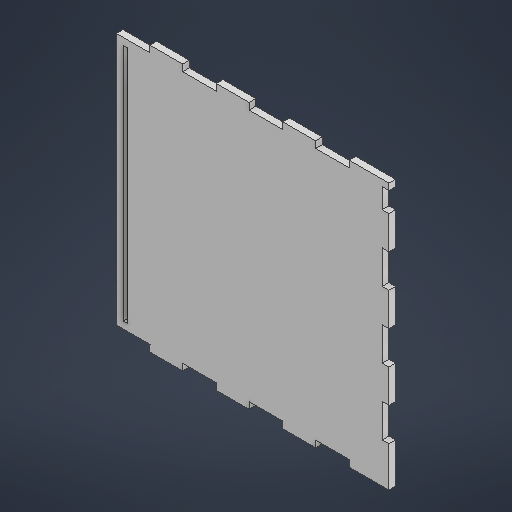
# Autodesk Inventor part: Base
Saved by Autodesk Inventor 2026 (Build 300175050, 175E)
## iProperties
Created: 2025-08-08
Part Number: Base
Material: Genérico
Document SubType Name: Modeling
Designer: EspacoMaker
Density: 1 g/cm^3
Appearance: Padrão
Author: EspacoMaker
Autodesk Inventor part; units mm, degrees
ref_plane "YZ Plane" through (0, 0, 0) normal (1, 0, 0) x (0, 1, 0)
ref_plane "XZ Plane" through (0, 0, 0) normal (0, 1, 0) x (-1, 0, 0)
ref_plane "XY Plane" through (0, 0, 0) normal (0, 0, 1) x (1, 0, 0)
sketch "Esboço1" plane through (0, 0, 0) normal (0, 0, 1) x (1, 0, 0)
  line L0 (-60, -60) -> (60, -60)
  line L1 (60, -60) -> (60, 60)
  line L2 (60, 60) -> (-60, 60)
  line L3 (-60, 60) -> (-60, -60)
  line L4 (-60, -60) -> (60, 60) construction
  line L5 (60, -60) -> (-60, 60) construction
  point P0 (0, 0)
  dimension "d0" = 120
  dimension "d1" = 120
  constraints: 12 end point, 2 midpoint, 2 parallel, 1 horizontal, 1 perpendicular
  measures "d0" distance of L2.end L1.end
  measures "d1" distance of L1.end L0.end
extrude "Extrusão1" add sketch "Esboço1" along normal blind 3
sketch "Esboço2" plane through (-60, 60, 0) normal (0, 1, 0) x (1, 0, 0)
  line L0 (120, -3) -> (0, -3) projected
  line L1 (120, 0) -> (0, 0) projected
  line L2 (0, -3) -> (15.1, -3)
  line L3 (15.1, -3) -> (15.1, 0)
  line L4 (15.1, 0) -> (0, 0)
  line L5 (0, 0) -> (0, -3)
  line L6 (-0.1, 0) -> (-0.1, -3)
  line L7 (29.9, 0) -> (29.9, -3)
  line L8 (45.1, 0) -> (30, 0)
  line L9 (30, -3) -> (45.1, -3)
  line L10 (45.1, -3) -> (45.1, 0)
  line L11 (59.9, 0) -> (59.9, -3)
  line L12 (75.1, 0) -> (60, 0)
  line L13 (60, -3) -> (75.1, -3)
  line L14 (75.1, -3) -> (75.1, 0)
  line L15 (89.9, 0) -> (89.9, -3)
  line L16 (105.1, 0) -> (90, 0)
  line L17 (90, -3) -> (105.1, -3)
  line L18 (105.1, -3) -> (105.1, 0)
  point P0 (89.9, 0)
  point P1 (59.9, 0)
  point P2 (29.9, 0)
  dimension "d4" = 15.1
  dimension "d57" = 30
  dimension "d63" = 0.1
  constraints: 34 end point, 9 point on line, 2 horizontal, 2 parallel, 2 perpendicular, 30 other
  measures "d4" distance of L4.end L3.end
  measures "d57" distance of L6.start L7.start
  measures "d63" distance between parallel lines of L6 L5
extrude "Extrusão2" cut sketch "Esboço2" against normal blind 3 contours L0 L15 L1 L18 | L0 L11 L1 L14 | L0 L7 L1 L10 | L0 L5 L1 L3
sketch "Esboço3" plane through (-60, -60, 0) normal (0, -1, 0) x (1, 0, 0)
  line L0 (0, 0) -> (120, 0) projected
  line L1 (0, 3) -> (15.1, 3)
  line L2 (15.1, 3) -> (15.1, 0)
  line L3 (15.1, 0) -> (0, 0)
  line L4 (0, 0) -> (0, 3)
  line L5 (-0.1, 0) -> (-0.1, 3)
  line L6 (-0.1, 0) -> (15.1, 0)
  line L7 (15.1, 0) -> (15.1, 3)
  line L8 (15.1, 3) -> (-0.1, 3)
  line L9 (-0.1, 3) -> (-0.1, 0)
  line L10 (29.9, 0) -> (29.9, 3)
  line L11 (45.1, 0) -> (30, 0)
  line L12 (30, 3) -> (45.1, 3)
  line L13 (45.1, 3) -> (45.1, 0)
  line L14 (59.9, 0) -> (59.9, 3)
  line L15 (75.1, 0) -> (60, 0)
  line L16 (60, 3) -> (75.1, 3)
  line L17 (75.1, 3) -> (75.1, 0)
  line L18 (89.9, 0) -> (89.9, 3)
  line L19 (105.1, 0) -> (90, 0)
  line L20 (90, 3) -> (105.1, 3)
  line L21 (105.1, 3) -> (105.1, 0)
  line L22 (0, 0) -> (0, 3) projected
  line L23 (0, 3) -> (120, 3) projected
  line L24 (120, 3) -> (120, 0) projected
  line L25 (120, 0) -> (0, 0) projected
  point P0 (-0.1, 1.5)
  point P1 (29.9, 1.5)
  point P2 (59.9, 1.5)
  point P3 (89.9, 1.5)
  point P4 (105.1, 0)
  point P5 (89.9, 0)
  point P6 (75.1, 0)
  point P7 (59.9, 0)
  point P8 (45.1, 0)
  point P9 (29.9, 0)
  dimension "d14" = 15.1
  dimension "d47" = 15.2
  dimension "d50" = 30
  dimension "d64" = 0.1
  constraints: 42 end point, 9 point on line, 4 parallel, 3 horizontal, 3 perpendicular, 1 collinear, 1 midpoint, 34 other
  measures "d14" distance of L2.end L3.end
  measures "d47" distance of L8.end L1.end
  measures "d50" distance of L5.start L10.start
  measures "d64" distance between parallel lines of L5 L4
extrude "Extrusão3" cut sketch "Esboço3" against normal blind 3 contours L4 L1 L2 L0 | L10 L23 L12 L13 L0 | L14 L23 L16 L17 L0 | L18 L23 L20 L21 L0
sketch "Esboço5" plane through (60, -60, 0) normal (1, 0, 0) x (0, 0, -1)
  line L0 (0, 3) -> (-3, 3) projected
  line L1 (-3, 3) -> (0, 3)
  line L2 (0, 3) -> (0, 18.1)
  line L3 (0, 18.1) -> (-3, 18.1)
  line L4 (-3, 18.1) -> (-3, 3)
  line L5 (0, 0) -> (-3, 0) projected
  line L6 (-3, 0) -> (-3, 120) projected
  line L7 (-3, 120) -> (0, 120) projected
  line L8 (0, 120) -> (0, 0) projected
  line L9 (0, 0) -> (-3, 0) projected
  line L10 (-3, 0) -> (-3, 120) projected
  line L11 (-3, 120) -> (0, 120) projected
  line L12 (0, 120) -> (0, 0) projected
  line L13 (-3, 3.1) -> (0, 3.1)
  line L14 (-3, 33.1) -> (0, 33.1)
  line L15 (0, 48.1) -> (-3, 48.1)
  line L16 (-3, 63.1) -> (0, 63.1)
  line L17 (0, 78.1) -> (-3, 78.1)
  line L18 (-3, 93.1) -> (0, 93.1)
  line L19 (0, 108.1) -> (-3, 108.1)
  line L20 (-3, 123.1) -> (0, 123.1)
  line L21 (0, 138.1) -> (-3, 138.1)
  line L22 (-3, 153.1) -> (0, 153.1)
  line L23 (0, 168.1) -> (-3, 168.1)
  line L24 (-3, 183.1) -> (0, 183.1)
  line L25 (0, 198.1) -> (-3, 198.1)
  line L26 (-3, 213.1) -> (0, 213.1)
  line L27 (0, 228.1) -> (-3, 228.1)
  line L28 (-3, 243.1) -> (0, 243.1)
  line L29 (0, 258.1) -> (-3, 258.1)
  line L30 (-3, 273.1) -> (0, 273.1)
  line L31 (0, 288.1) -> (-3, 288.1)
  line L32 (-3, 117.1) -> (0, 117.1)
  point P0 (-1.5, 3)
  point P1 (-3, 3.1)
  point P2 (-1.5, 120)
  dimension "d35" = 3
  dimension "d36" = 15.1
  dimension "d65" = 0.1
  dimension "d68" = 30
  dimension "d73" = 2.9
  constraints: 48 end point, 4 point on line, 3 perpendicular, 2 midpoint, 2 parallel, 1 horizontal, 1 vertical, 54 other
  measures "d35" distance of L3.end L2.end
  measures "d36" distance of L2.end L1.end
  measures "d65" distance from line of L13 point (-1.5, 3)
  measures "d68" distance of L13.start L14.start
  measures "d73" distance from line of L32 point (-1.5, 120)
extrude "Extrusão5" add sketch "Esboço5" along normal blind 3 contours L8 L5 L6 L0 | L0 L4 L13 L2 | L13 L4 L3 L2 | L14 L6 L15 L8 | L16 L6 L17 L8 | L18 L6 L19 L8 | L32 L6 L7 L8
sketch "Esboço6" plane through (0, 0, 3) normal (0, 0, 1) x (1, 0, 0)
  line L0 (-54.8, -53.9) -> (-57, -53.9)
  line L1 (-57, -53.9) -> (-57, 53.9)
  line L2 (-57, 53.9) -> (-54.8, 53.9)
  line L3 (-54.8, 53.9) -> (-54.8, -53.9)
  line L4 (-54.8, -53.9) -> (-57, 53.9) construction
  line L5 (-57, -53.9) -> (-54.8, 53.9) construction
  line L6 (-44.9, 57) -> (-60, 57) projected
  line L7 (-60, 57) -> (-60, -57) projected
  point P0 (0, 0)
  point P1 (-55.9, 0)
  dimension "d74" = 3.1
  dimension "d75" = 3
  dimension "d76" = 2.2
  constraints: 12 end point, 2 midpoint, 2 parallel, 1 horizontal, 1 horizontal alignment, 1 perpendicular
  measures "d74" distance between parallel lines of L6 L2
  measures "d75" distance between parallel lines of L7 L1
  measures "d76" distance between parallel lines of L1 L3
extrude "Extrusão6" cut sketch "Esboço6" against normal up to surface (3 mm away)
